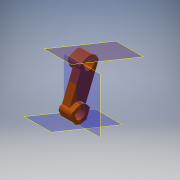
# Autodesk Inventor part: HbRing-LittleCouplerLink01
Saved by Autodesk Inventor 2017 (Build 210142000, 142)
## iProperties
Created: 2015-02-23
Part Number: HbRing-LittleCouplerLink01
Material: ナイロン 6/6
Document SubType Name: Modeling
Designer: Yamaura
Density: 1.13 g/cm^3
Appearance: 滑らか - 淡いオレンジ
Author: Yamaura
Autodesk Inventor part; units mm, degrees
ref_plane "YZ Plane" through (0, 0, 0) normal (1, 0, 0) x (0, 1, 0)
ref_plane "XY Plane" through (0, 0, 0) normal (0, 0, 1) x (1, 0, 0)
sketch "スケッチ1" plane through (0, 0, 0) normal (1, 0, 0) x (0, 1, 0)
  arc A0 (-2.7792, 1.1297) -> (2.7792, -1.1297) centre (0, 0) ccw
  circle A1 centre (5, 12.3) radius 1.7
  arc A2 (7.7792, 11.1703) -> (2.2208, 13.4297) centre (5, 12.3) ccw
  circle A3 centre (0, 0) radius 1.7
  line L0 (2.2208, 13.4297) -> (-2.7792, 1.1297)
  line L1 (7.7792, 11.1703) -> (2.7792, -1.1297)
  dimension "d1" = 3.4
  dimension "d2" = 6
  dimension "d3" = 3.4
  dimension "d4" = 5
  dimension "d5" = 12.3
  dimension "d8" = 3
  constraints: 4 centre point, 4 end point, 4 point on circle, 4 tangent, 3 coincident
  measures "d1" diameter of A1
  measures "d2" diameter of A2
  measures "d3" diameter of A3
  measures "d4" horizontal distance of A1.centre point (0, 0)
  measures "d5" vertical distance of A1.centre point (0, 0)
  measures "d8" radius of A0
extrude "押し出し1" add sketch "スケッチ1" against normal blind 6.2
sketch "スケッチ2" plane through (0, 0, 0) normal (1, 0, 0) x (0, 0, -1)
  circle A0 centre (0, 0) radius 1.7 projected
  circle A1 centre (-12.3, 5) radius 1.7 projected
  line L0 (-1.1297, -2.7792) -> (-13.4297, 2.2208) projected
  arc A2 (-1.1297, -2.7792) -> (1.1297, 2.7792) centre (0, 0) ccw projected
  line L1 (-11.1703, 7.7792) -> (1.1297, 2.7792) projected
  arc A3 (-11.1703, 7.7792) -> (-13.4297, 2.2208) centre (-12.3, 5) ccw projected
  circle A4 centre (0, 0) radius 3
  line L2 (-1.1297, -2.7792) -> (1.1297, 2.7792)
  dimension "d11" = 6
  constraints: 2 end point, 1 coincident, 1 midpoint, 1 perpendicular, 1 point on line, 3 other
extrude "押し出し2" cut sketch "スケッチ2" against normal blind 1.7 contours A4 L0 A3 L1
sketch "スケッチ3" plane through (-6.2, 0, 0) normal (-1, 0, 0) x (0, 0, 1)
  circle A0 centre (0, 0) radius 1.7 projected
  circle A1 centre (12.3, 5) radius 1.7 projected
  line L0 (1.1297, -2.7792) -> (13.4297, 2.2208) projected
  arc A2 (13.4297, 2.2208) -> (11.1703, 7.7792) centre (12.3, 5) ccw projected
  line L1 (11.1703, 7.7792) -> (-1.1297, 2.7792) projected
  arc A3 (-1.1297, 2.7792) -> (1.1297, -2.7792) centre (0, 0) ccw projected
  circle A4 centre (12.3, 5) radius 3
  line L2 (11.1703, 7.7792) -> (13.4297, 2.2208)
  line L3 (1.1297, -2.7792) -> (13.4297, 2.2208) projected
  dimension "d14" = 6
  constraints: 2 end point, 1 coincident, 1 midpoint, 1 perpendicular, 1 point on line, 3 other
extrude "押し出し3" cut sketch "スケッチ3" against normal blind 1.7 contours A4 L0 A3 L1
sketch "スケッチ4" plane through (-1.7, 0, 0) normal (1, 0, 0) x (0, 0, -1)
  arc A0 (1.1297, 2.7792) -> (-1.1297, -2.7792) centre (0, 0) ccw projected
  line L0 (-11.1703, 7.7792) -> (1.1297, 2.7792) projected
  arc A1 (-11.1703, 7.7792) -> (-13.4297, 2.2208) centre (-12.3, 5) ccw projected
  line L1 (-1.1297, -2.7792) -> (-13.4297, 2.2208) projected
  circle A2 centre (-12.3, 5) radius 1.7 projected
  line L2 (-13.4297, 2.2208) -> (-13.8977, 1.0697)
  line L3 (-13.8977, 1.0697) -> (-15.064, 3.8337)
  arc A3 (-11.1703, 7.7792) -> (-13.4297, 2.2208) centre (-12.3, 5) ccw projected
  dimension "d17" = 45
  constraints: 4 end point, 1 perpendicular, 1 point on circle, 1 point on line, 1 tangent
  measures "d17" angle of L3 L2
extrude "押し出し4" add sketch "スケッチ4" against normal up to surface (4.5 mm away) contours L2 L3 A1
mirror "ミラー1" about plane through (-1.7, 2.2208, 13.4297) normal (0, -0.3765791, -0.9263845) of "押し出し4"
sketch "スケッチ5" plane through (-1.7, 0, 0) normal (1, 0, 0) x (0, 0, -1)
  line L0 (-1.1297, -2.7792) -> (-12.2786, 1.7529) projected
  arc A0 (1.1297, 2.7792) -> (-1.1297, -2.7792) centre (0, 0) ccw projected
  line L1 (-11.1703, 7.7792) -> (1.1297, 2.7792) projected
  arc A1 (-11.1703, 7.7792) -> (-15.064, 3.8337) centre (-12.3, 5) ccw projected
  line L2 (-15.064, 3.8337) -> (-13.8977, 1.0697) projected
  line L3 (-12.2786, 1.7529) -> (-13.8977, 1.0697) projected
  circle A2 centre (-12.3, 5) radius 1.7 projected
  line L4 (-12.9402, 3.4251) -> (-13.2054, 2.7728)
  line L5 (-13.2054, 2.7728) -> (-13.8663, 4.3391)
  circle A3 centre (-12.3, 5) radius 1.7 projected
  arc A4 (-13.8663, 4.3391) -> (-12.9402, 3.4251) centre (-12.3, 5) ccw
  dimension "d20" = 45
  constraints: 4 end point, 2 point on circle, 1 centre point, 1 coincident, 1 perpendicular, 3 other
  measures "d20" angle of L5 L4
extrude "押し出し5" cut sketch "スケッチ5" against normal blind 10 contours A2 L4 L5
mirror "ミラー2" about plane through (-1.7, 3.4251, 12.9402) normal (0, 0.3765791, 0.9263845) of "押し出し5"
fillet "フィレット1" radius 1.3 1 edges at (-3.95, 1.0697, 13.8977)
sketch "スケッチ6" plane through (-4.5, 0, 0) normal (-1, 0, 0) x (0, 0, 1)
  circle A0 centre (0, 0) radius 1.7 projected
  line L0 (12.2786, 1.7529) -> (11.1337, 2.236) projected
  arc A1 (11.1703, 7.7792) -> (11.1337, 2.236) centre (12.3, 5) ccw projected
  line L1 (-1.1297, 2.7792) -> (11.1703, 7.7792) projected
  arc A2 (-1.1297, 2.7792) -> (1.1297, -2.7792) centre (0, 0) ccw projected
  line L2 (12.2786, 1.7529) -> (1.1297, -2.7792) projected
  line L3 (1.1297, -2.7792) -> (1.5977, -3.9303)
  line L4 (1.5977, -3.9303) -> (-1.1663, -2.764)
  dimension "d24" = 45
  constraints: 4 end point, 1 perpendicular, 1 point on circle, 1 point on line, 1 tangent
  measures "d24" angle of L4 L3
extrude "押し出し6" add sketch "スケッチ6" against normal up to surface (4.5 mm away) contours L3 L4 A2
mirror "ミラー3" about plane through (-4.5, -2.7792, 1.1297) normal (0, 0.3765791, 0.9263845) of "押し出し6"
sketch "スケッチ7" plane through (-4.5, 0, 0) normal (-1, 0, 0) x (0, 0, 1)
  circle A0 centre (0, 0) radius 1.7 projected
  line L0 (0.6402, -1.5749) -> (0.9054, -2.2272)
  line L1 (0.9054, -2.2272) -> (-0.6609, -1.5663)
  line L2 (-1.1297, 2.7792) -> (11.1703, 7.7792) projected
  dimension "d29" = 45
  constraints: 4 end point, 2 point on circle, 1 perpendicular, 1 tangent
  measures "d29" angle of L1 L0
extrude "押し出し7" cut sketch "スケッチ7" against normal blind 10 contours A0 L0 L1
mirror "ミラー4" about plane through (-4.5, -1.5749, 0.6402) normal (0, -0.3765791, -0.9263845) of "押し出し7"
fillet "フィレット2" radius 1.3 1 edges at (-2.25, -3.9303, 1.5977)
sketch "スケッチ8" plane through (-4.5, 0, 0) normal (-1, 0, 0) x (0, 0, 1)
  line L0 (-1.1297, 2.7792) -> (11.1703, 7.7792) projected
  arc A0 (-1.1297, 2.7792) -> (-1.1663, -2.764) centre (0, 0) ccw projected
  line L1 (-1.1297, 2.7792) -> (-2.7291, 2.129)
  line L2 (-2.7291, 2.129) -> (-2.9705, 0.4196)
  constraints: 4 end point, 1 collinear, 1 point on circle, 1 tangent
extrude "押し出し8" add sketch "スケッチ8" against normal up to surface (4.5 mm away)
ref_plane "作業平面1" through (0, 2.7792, -1.1297) normal (0, -0.3765791, -0.9263845) x (-1, 0, 0)
mirror "ミラー5" about plane through (0, 2.7792, -1.1297) normal (0, -0.3765791, -0.9263845) of "押し出し8"
sketch "スケッチ9" plane through (-6.2, 0, 0) normal (-1, 0, 0) x (0, 0, 1)
  arc A0 (12.7, 1.5751) -> (14.4031, 2.2674) centre (13.2054, 2.7728) ccw projected
  line L0 (14.4031, 2.2674) -> (15.064, 3.8337) projected
  arc A1 (15.064, 3.8337) -> (11.1337, 2.236) centre (12.3, 5) ccw projected
  line L1 (12.7, 1.5751) -> (11.1337, 2.236) projected
  line L2 (13.2054, 2.7728) -> (11.6391, 3.4337) projected
  arc A2 (13.8663, 4.3391) -> (11.6391, 3.4337) centre (12.3, 5) ccw projected
  line L3 (13.8663, 4.3391) -> (13.2054, 2.7728) projected
  line L4 (-2.7291, 2.129) -> (11.1703, 7.7792) projected
  line L5 (11.1703, 7.7792) -> (12.4648, 8.3054)
  line L6 (12.4648, 8.3054) -> (13.7006, 7.653)
  point P0 (0, 0)
  constraints: 4 end point, 1 collinear, 1 point on circle, 1 tangent
extrude "押し出し9" add sketch "スケッチ9" against normal up to surface (4.5 mm away) contours L5 L6 A1
ref_plane "作業平面2" through (0, 7.7792, 11.1703) normal (0, -0.3765791, -0.9263845) x (-1, 0, 0)
mirror "ミラー6" about plane through (0, 7.7792, 11.1703) normal (0, -0.3765791, -0.9263845) of "押し出し9"
ref_plane "作業平面3" through (0, 7.7792, 11.1703) normal (0, -0.3765791, -0.9263845) x (-1, 0, 0)
scale "尺度2" factors (0.69, 0.69, 0.69) then translate (-1.395, -0.0865, 2.2567) bodies 1
